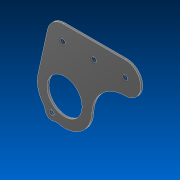
# Autodesk Inventor part: Intake Joint Holder Using 1__16 Gray Tinted Polycarbonate Sheet (36 x 72) (217-6627)
Saved by Autodesk Inventor 2022.2 (Build 262287000, 287)
## iProperties
Created: 2022-01-11
Part Number: Intake Joint Holder Using 1__16 Gray Tinted Polycarbonate Sheet (36 x 72) (217-6627)
Material: Polycarbonate, Clear
Document SubType Name: Modeling
Designer: omard
Density: 1.2 g/cm^3
Appearance: Smooth - Black
Author: omard
Autodesk Inventor part; units mm, degrees
ref_plane "YZ Plane" through (0, 0, 0) normal (1, 0, 0) x (0, 1, 0)
ref_plane "XZ Plane" through (0, 0, 0) normal (0, 1, 0) x (-1, 0, 0)
ref_plane "XY Plane" through (0, 0, 0) normal (0, 0, 1) x (1, 0, 0)
sketch "Sketch1" plane through (0, 0, 0) normal (0, 0, 1) x (1, 0, 0)
  circle A0 centre (0, 0) radius 14.2875
  circle A1 centre (-1.4096, 37.9321) radius 2.0701
  circle A2 centre (23.9904, 37.9321) radius 2.0701
  circle A3 centre (49.3904, 37.9321) radius 2.0701
  line L0 (-1.4096, 37.9321) -> (49.3904, 37.9321) construction
  circle A4 centre (0, 0) radius 22.225
  line L1 (-1.4096, 37.9321) -> (49.3904, 37.9321) construction
  line L2 (-1.4096, 25.2321) -> (49.3904, 25.2321) construction
  line L3 (49.3904, 50.6321) -> (-1.4096, 50.6321)
  arc A5 (-1.4096, 50.6321) -> (-1.4096, 25.2321) centre (-1.4096, 37.9321) ccw
  arc A6 (49.3904, 25.2321) -> (49.3904, 50.6321) centre (49.3904, 37.9321) ccw
  line L4 (-21.7062, 4.7742) -> (-13.8131, 40.6603)
  arc A7 (49.3904, 25.2321) -> (22.2073, -0.887) centre (49.3904, -1.9727) ccw
  line L5 (-10.67, -20.3) -> (-13.7684, -18.3404) construction
  line L6 (-13.7684, -18.3404) -> (-13.6206, -14.6772) construction
  line L7 (-13.6206, -14.6772) -> (-10.3742, -12.9737) construction
  line L8 (-10.3742, -12.9737) -> (-7.2757, -14.9333) construction
  line L9 (-7.2757, -14.9333) -> (-7.4236, -18.5965) construction
  line L10 (-7.4236, -18.5965) -> (-10.67, -20.3) construction
  circle A8 centre (0, 0) radius 16.51 construction
  circle A9 centre (-10.5221, -16.6369) radius 2.0701
  line L11 (-10.5221, -16.6369) -> (0, 0) construction
  circle A10 centre (-10.5221, -16.6369) radius 5.3975
  arc A11 (-15.8971, -17.1289) -> (-17.1155, -14.1778) centre (-21.2721, -17.621) ccw
  arc A12 (-5.4746, -21.5402) -> (-8.6631, -21.7041) centre (-6.8041, -26.7714) ccw
  circle A13 centre (-10.5221, -16.6369) radius 4.0005 construction
  point P0 (23.9904, 37.9321)
  point P1 (-12.2192, -19.3202)
  dimension "d0" = 25.4
  dimension "d2" = 62.2757
  dimension "d3" = 37.9583
  dimension "d4" = 4.1402
  dimension "d5" = 28.575
  dimension "d6" = 44.45
  dimension "d7" = 25.4
  dimension "d10" = 6.35
  dimension "d11" = 33.02
  dimension "d12" = 8.001
  constraints: 26 end point, 17 point on circle, 14 centre point, 14 tangent, 6 coincident, 5 equal radius, 3 midpoint, 2 equal length, 1 horizontal, 1 perpendicular, 1 point on line, 13 other
  measures "d0" distance of A2.centre L0.start
  measures "d2" distance of L0.end point (0, 0)
  measures "d3" distance of point (0, 0) L0.start
  measures "d4" diameter of A1
  measures "d5" diameter of A0
  measures "d6" diameter of A4
  measures "d7" diameter of A6
  measures "d10" distance from line of point (-12.219, -19.32) L8
  measures "d11" diameter of A8
  measures "d12" diameter of A13
extrude "Extrusion1" add sketch "Sketch1" along normal blind 1.5875
body "Solid1"
